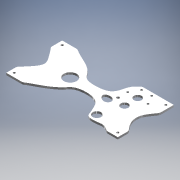
# Autodesk Inventor part: V2 Plate 1
Saved by Autodesk Inventor 2019.4 (Build 234330000, 330)
## iProperties
Created: 2020-03-11
Part Number: V2 Plate 1
Material: Aluminum 6061
Document SubType Name: Modeling
Designer: Mark
Mass: 501.631 g
Surface Area: 806.098 cm^2
Volume: 185.789 cm^3
Density: 2.7 g/cm^3
Appearance: Aluminum - Flat
Author: Mark
Autodesk Inventor part; units mm, degrees
ref_plane "YZ Plane" through (0, 0, 0) normal (1, 0, 0) x (0, 1, 0)
ref_plane "XZ Plane" through (0, 0, 0) normal (0, 1, 0) x (-1, 0, 0)
ref_plane "XY Plane" through (0, 0, 0) normal (0, 0, 1) x (1, 0, 0)
sketch "Sketch1" plane through (0, 0, 0) normal (0, 1, 0) x (-1, 0, 0)
  line L0 (0, 0) -> (279, 0)
  line L1 (279, 0) -> (279, -140)
  line L2 (279, -140) -> (0, -140)
  line L3 (0, -140) -> (0, 0)
  circle A0 centre (10, -10) radius 2.75
  circle A1 centre (10, -130) radius 2.75
  circle A2 centre (269, -10) radius 2.75
  circle A3 centre (269, -130) radius 2.75
  dimension "d0" = 279
  dimension "d1" = 140
  dimension "d2" = 5.5
  dimension "d3" = 5.5
  dimension "d4" = 5.5
  dimension "d5" = 5.5
  dimension "d6" = 10
  dimension "d7" = 10
  dimension "d8" = 10
  dimension "d9" = 10
  dimension "d10" = 10
  dimension "d11" = 10
  dimension "d12" = 10
  dimension "d13" = 10
  constraints: 8 end point, 4 centre point, 2 parallel, 1 horizontal, 1 perpendicular
  measures "d0" distance of L1.end L2.end
  measures "d1" distance of L0.end L1.end
  measures "d2" diameter of A0
  measures "d3" diameter of A1
  measures "d4" diameter of A2
  measures "d5" diameter of A3
  measures "d6" distance from line of L2 A3.centre
  measures "d7" distance from line of L1 A3.centre
  measures "d8" distance from line of L1 A2.centre
  measures "d9" distance from line of L0 A2.centre
  measures "d10" distance from line of L3 A0.centre
  measures "d11" distance from line of A0.centre L0
  measures "d12" distance from line of L3 A1.centre
  measures "d13" distance from line of L2 A1.centre
extrude "Extrusion1" add sketch "Sketch1" along normal blind 5
sketch "Sketch2" plane through (0, 0, 0) normal (0, -1, 0) x (1, 0, 0)
  circle A0 centre (-60, -110) radius 9.575
  line L0 (-279, -140) -> (0, -140) projected
  line L1 (0, -140) -> (0, 0) projected
  line L2 (-60, -110) -> (-60, -76.98) construction
  circle A1 centre (-60, -76.98) radius 9.5
  circle A2 centre (-60, -110) radius 25.4 construction
  circle A3 centre (-34.6, -110) radius 2.6
  circle A4 centre (-60, -110) radius 25.4 construction
  circle A5 centre (-47.3, -88.003) radius 2.6
  circle A6 centre (-60, -110) radius 25.4 construction
  circle A7 centre (-72.7, -88.003) radius 2.6
  circle A8 centre (-60, -110) radius 25.4 construction
  circle A9 centre (-85.4, -110) radius 2.6
  circle A10 centre (-60, -110) radius 25.4 construction
  circle A11 centre (-72.7, -131.997) radius 2.6
  circle A12 centre (-60, -110) radius 25.4 construction
  circle A13 centre (-47.3, -131.997) radius 2.6
  line L3 (-60, -110) -> (-59, -110) construction
  line L4 (-60, -110) -> (-30, -110) construction
  line L5 (-60, -110) -> (-30, -110) construction
  circle A14 centre (-75, -22.7669) radius 10.5
  line L6 (-60, -76.98) -> (-75, -22.7669) construction
  line L7 (-75, -22.7669) -> (-188.9701, -70) construction
  line L8 (-279.0043, -70) -> (0, -70) construction
  line L9 (0, 0) -> (0, -140) projected
  circle A15 centre (-188.9701, -70) radius 16
  dimension "d23" = 50.8
  dimension "d16" = 19.15
  dimension "d17" = 30
  dimension "d18" = 60
  dimension "d19" = 33.02
  dimension "d20" = 19
  dimension "d24" = 5.2
  dimension "d27" = 360
  dimension "d31" = 30
  dimension "d32" = 0
  dimension "d33" = 21
  dimension "d34" = 56.25
  dimension "d35" = 15
  dimension "d36" = 123.37
  dimension "d37" = 32
  constraints: 14 end point, 10 centre point, 4 coincident, 2 horizontal, 2 horizontal alignment, 2 parallel, 2 point on line, 1 collinear, 1 midpoint, 41 other
  measures "d16" diameter of A0
  measures "d17" distance from line of L0 L2.start
  measures "d18" distance from line of L1 L2.start
  measures "d19" distance of L2.start L2.end
  measures "d20" diameter of A1
  measures "d24" diameter of A3
  measures "d31" distance of L3.start L4.end
  measures "d32" distance between parallel lines of L4 L5
  measures "d33" diameter of A14
  measures "d34" distance of L6.start L6.end
  measures "d35" horizontal distance of L6.start A14.centre
  measures "d36" distance of L6.end L7.end
  measures "d37" diameter of A15
extrude "Extrusion2" cut sketch "Sketch2" against normal blind 5 contours A0 | A1 | A3 | A9 | A11 | A13 | A14 | A15
sketch "Sketch3" plane through (0, 5, 0) normal (0, 1, 0) x (1, 0, 0)
  line L0 (-279, 110.51) -> (-275.673, 108.913) construction
  line L1 (-275.673, 108.913) -> (-264.4231, 92.7718) construction
  line L2 (-264.4231, 92.7718) -> (-250.8906, 76.3046) construction
  line L3 (-250.8906, 76.3046) -> (-249.2602, 64.0765) construction
  line L4 (-249.2602, 64.0765) -> (-255.6188, 53.6418) construction
  line L5 (-255.6188, 53.6418) -> (-264.9122, 41.7397) construction
  line L6 (-279, 140) -> (-279, 0) projected
  line L7 (-264.9122, 41.7397) -> (-279, 26.3127) construction
  spline S0 degree 4 poles (-279, 110.51) (-275.673, 108.913) (-264.4231, 92.7718) (-250.8906, 76.3046) (-249.2602, 64.0765) (-255.6188, 53.6418) (-264.9122, 41.7397) (-279, 26.3127) knots 1 1 1 1 1 2 3 4 5 5 5 5 5
  line L8 (-240.8569, 140) -> (-226.9801, 130.8595) construction
  line L9 (-226.9801, 130.8595) -> (-202.6636, 121.4616) construction
  line L10 (-202.6636, 121.4616) -> (-183.7353, 109.7282) construction
  line L11 (-183.7353, 109.7282) -> (-174.006, 97.889) construction
  line L12 (-174.006, 97.889) -> (-165.4012, 82.5088) construction
  line L13 (-165.4012, 82.5088) -> (-130.5867, 82.5088) construction
  line L14 (-130.5867, 82.5088) -> (-105.3862, 87.3158) construction
  line L15 (-105.3862, 87.3158) -> (-97.3745, 106.9809) construction
  line L16 (-97.3745, 106.9809) -> (-96.3549, 122.1303) construction
  line L17 (-96.3549, 122.1303) -> (-88.7207, 131.9075) construction
  line L18 (0, 140) -> (-279, 140) projected
  line L19 (-88.7207, 131.9075) -> (-78.8731, 140) construction
  spline S1 degree 4 poles (-240.8569, 140) (-226.9801, 130.8595) (-202.6636, 121.4616) (-183.7353, 109.7282) (-174.006, 97.889) (-165.4012, 82.5088) (-130.5867, 82.5088) (-105.3862, 87.3158) (-97.3745, 106.9809) (-96.3549, 122.1303) (-88.7207, 131.9075) (-78.8731, 140) knots 1 1 1 1 1 2 3 4 5 6 7 8 9 9 9 9 9
  line L20 (-236.648, 0) -> (-234.4713, 3.3996) construction
  line L21 (-234.4713, 3.3996) -> (-211.7179, 14.0237) construction
  line L22 (-211.7179, 14.0237) -> (-188.9329, 27.3145) construction
  line L23 (-188.9329, 27.3145) -> (-171.6954, 43.2741) construction
  line L24 (-171.6954, 43.2741) -> (-166.204, 55.3552) construction
  line L25 (-166.204, 55.3552) -> (-133.7615, 60.8756) construction
  line L26 (-133.7615, 60.8756) -> (-103.4379, 53.6418) construction
  line L27 (-103.4379, 53.6418) -> (-95.2388, 35.218) construction
  line L28 (-95.2388, 35.218) -> (-86.7794, 17.4074) construction
  line L29 (-86.7794, 17.4074) -> (-85.5108, 9.5701) construction
  line L30 (-85.5108, 9.5701) -> (-77.1088, 6.3107) construction
  line L31 (-77.1088, 6.3107) -> (-62.7675, 6.3107) construction
  line L32 (-62.7675, 6.3107) -> (-52.4824, 8.5561) construction
  line L33 (-52.4824, 8.5561) -> (-45.5652, 9.208) construction
  line L34 (-45.5652, 9.208) -> (-35.9319, 6.347) construction
  line L35 (-35.9319, 6.347) -> (-29.8656, 1.6103) construction
  line L36 (-29.8656, 1.6103) -> (-29.8656, 0) construction
  spline S2 degree 4 poles (-236.648, 0) (-234.4713, 3.3996) (-211.7179, 14.0237) (-188.9329, 27.3145) (-171.6954, 43.2741) (-166.204, 55.3552) (-133.7615, 60.8756) (-103.4379, 53.6418) (-95.2388, 35.218) (-86.7794, 17.4074) (-85.5108, 9.5701) (-77.1088, 6.3107) (-62.7675, 6.3107) (-52.4824, 8.5561) (-45.5652, 9.208) (-35.9319, 6.347) (-29.8656, 1.6103) (-29.8656, 0) knots 1 1 1 1 1 2 3 4 5 6 7 8 9 10 11 12 13 14 15 15 15 15 15
  line L37 (-91.0091, 78.3089) -> (-99.8286, 80.9282) construction
  line L38 (-99.8286, 80.9282) -> (-111.7701, 77.1363) construction
  line L39 (-111.7701, 77.1363) -> (-111.7701, 68.319) construction
  line L40 (-111.7701, 68.319) -> (-98.2066, 58.1154) construction
  line L41 (-98.2066, 58.1154) -> (-86.7794, 60.232) construction
  line L42 (-86.7794, 60.232) -> (-82.336, 71.7291) construction
  line L43 (-82.336, 71.7291) -> (-91.0091, 78.3089) construction
  spline S3 degree 4 poles (-91.0091, 78.3089) (-99.8286, 80.9282) (-111.7701, 77.1363) (-111.7701, 68.319) (-98.2066, 58.1154) (-86.7794, 60.232) (-82.336, 71.7291) (-91.0091, 78.3089) knots 1 1 1 1 1 2 3 4 5 5 5 5 5
  line L44 (-279, 0) -> (0, 0) projected
  line L45 (0, 0) -> (0, 140) projected
  line L46 (0, 105.1152) -> (-13.7481, 85.7692) construction
  line L47 (-13.7481, 85.7692) -> (-22.7694, 71.7291) construction
  line L48 (-22.7694, 71.7291) -> (-19.2602, 53.6418) construction
  line L49 (-19.2602, 53.6418) -> (-11.755, 40.227) construction
  line L50 (-11.755, 40.227) -> (0, 27.4329) construction
  spline S4 degree 4 poles (0, 105.1152) (-13.7481, 85.7692) (-22.7694, 71.7291) (-19.2602, 53.6418) (-11.755, 40.227) (0, 27.4329) knots 1 1 1 1 1 2 3 3 3 3 3
  constraints: 6 point on line, 1 horizontal, 1 parallel, 1 vertical, 14 other
extrude "Extrusion3" cut sketch "Sketch3" against normal through all contours S0 L6 | L18 S1 | S2 L44 | L45 S4 | S3
fillet "Fillet1" radius 10 8 edges at (-240.8569, 2.5, -140) (-78.8731, 2.5, -140) (-279, 2.5, -26.3127) (-279, 2.5, -110.51) (-29.8656, 2.5, 0) (-236.648, 2.5, 0) (0, 2.5, -27.4329) (0, 2.5, -105.1152)
sketch "Sketch4" plane through (0, 0, 0) normal (0, -1, 0) x (1, 0, 0)
  circle A0 centre (-85.4091, -85.8895) radius 3.4
  circle A1 centre (-60, -76.98) radius 9.5 projected
  point P0 (0, 0)
  dimension "d43" = 6.8
  dimension "d44" = 25.4091
  dimension "d45" = 8.9095
  constraints: 1 centre point
  measures "d43" diameter of A0
  measures "d44" horizontal distance of A1.centre A0.centre
  measures "d45" vertical distance of A1.centre A0.centre
extrude "Extrusion4" cut sketch "Sketch4" against normal through all contours A0
body "Solid1"
